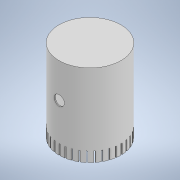
# Autodesk Inventor part: shroud
Saved by Autodesk Inventor 2020 (Build 240168000, 168)
## iProperties
Created: 2019-07-17
Part Number: shroud
Material: Generic
Document SubType Name: Modeling
Designer: ColinP
Density: 1 g/cm^3
Appearance: Default
Mass: 23.8561 g
Surface Area: 320.645 cm^2
Volume: 23.8561 cm^3
Author: ColinP
Autodesk Inventor part; units mm, degrees
ref_plane "YZ Plane" through (0, 0, 0) normal (1, 0, 0) x (0, 1, 0)
ref_plane "XZ Plane" through (0, 0, 0) normal (0, 1, 0) x (-1, 0, 0)
ref_plane "XY Plane" through (0, 0, 0) normal (0, 0, 1) x (1, 0, 0)
sketch "Sketch23" plane through (0, 0, 0) normal (0, 1, 0) x (-1, 0, 0)
  circle A0 centre (0, 0) radius 38.1
  circle A1 centre (0, 0) radius 39.37
  dimension "d82" = 76.2
  dimension "d83" = 78.74
  constraints: 2 centre point, 2 coincident
  measures "d82" diameter of A0
  measures "d83" diameter of A1
extrude "Extrusion14" add sketch "Sketch23" along normal blind 101.6
sketch "Sketch24" plane through (0, 101.6, 0) normal (0, 1, 0) x (1, 0, 0)
  circle A0 centre (0, 0) radius 38.1 projected
  circle A1 centre (0, 0) radius 39.37 projected
extrude "Extrusion15" add sketch "Sketch24" along normal blind 2.54 contours A0 | A1
sketch "Sketch30" plane through (0, 0, 0) normal (0, 0, 1) x (1, 0, 0)
  line L0 (0, 0) -> (0, 60.325)
  circle A0 centre (0, 60.325) radius 6.35
  dimension "d94" = 60.325
  dimension "d95" = 12.7
  constraints: 2 end point, 1 centre point, 1 coincident, 1 vertical
  measures "d94" distance of L0.start L0.end
  measures "d95" diameter of A0
extrude "Extrusion18" cut sketch "Sketch30" along normal mid plane 406.4
sketch "Sketch31" plane through (0, 0, 0) normal (0, -1, 0) x (1, 0, 0)
  circle A0 centre (0, 0) radius 39.37 projected
  arc A1 (-39.346, 1.374) -> (-39.37, 0) centre (0, 0) ccw
  line L0 (0, 0) -> (-39.346, 1.374) construction
  line L1 (0, 0) -> (-39.37, 0) construction
  circle A2 centre (0, 0) radius 38.1
  line L2 (-39.346, 1.374) -> (-38.0768, 1.3297)
  circle A3 centre (0, 0) radius 38.1 projected
  line L3 (-39.37, 0) -> (-38.1, 0)
  dimension "d98" = 2
  constraints: 8 end point, 5 point on circle, 2 centre point, 2 coincident, 2 point on line
  measures "d98" angle of L0 L1
extrude "Extrusion19" cut sketch "Sketch31" against normal blind 12.7 contours L2 A2 L3 A0 picked at (-38.9458, 0.1527)
pattern_circular "Circular Pattern3" count 36 over 360 about axis through (0, 0, 0) along (0, 1, 0) of "Extrusion19"
body "Solid4"
